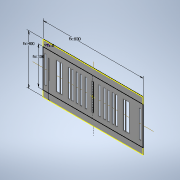
# Autodesk Inventor part: ferrite_layer_dex_1R1
Saved by Autodesk Inventor 2021 (Build 250183000, 183)
## iProperties
Created: 2021-01-27
Part Number: ferrite_layer_dex_1R1
Material: Generic
Document SubType Name: Modeling
Designer: pduy110
Density: 1 g/cm^3
Appearance: Smooth - Medium Gray
track_length: 800.000 mm
track_width: 300.000 mm
layer_width: 400.000 mm
ferrite_length: 218.000 mm
layer_length: 800.000 mm
real_sheet_width: 500.000 mm
ferrite_width: 15.000 mm
ferrite_height: 8.000 mm
number_of_ferrites: 7.000 ul
edge_gap_distance: 14.500 mm
parameter_2: 30.000 mm
parameter_5: 126.000 mm
parameter_6: 120.000 mm
bolt_diameter: 8.000 mm
number_of_bolts: 5.000 ul
x_offset_for_bolts: 75.000 mm
y_offset_for_bolts: 175.000 mm
wire_diameter: 4.500 mm
distance_between_wires: 18.600 mm
distance_between_wires_edge: 8.250 mm
bend_radius_inner: 15.000 mm
bend_radius_outer: 18.500 mm
wall_length: 800.000 mm
wall_width: 50.000 mm
wall_thickness: 25.000 mm
Author: pduy110
Autodesk Inventor part; units mm, degrees
ref_plane "YZ Plane" through (0, 0, 0) normal (1, 0, 0) x (0, 1, 0)
ref_plane "XZ Plane" through (0, 0, 0) normal (0, 1, 0) x (-1, 0, 0)
ref_plane "XY Plane" through (0, 0, 0) normal (0, 0, 1) x (1, 0, 0)
sketch "ferrite_layer_outline_sketch" plane through (0, 0, 0) normal (0, 0, 1) x (1, 0, 0)
  line L0 (-400, 200) -> (400, 200)
  line L1 (400, 200) -> (400, -200)
  line L2 (400, -200) -> (-400, -200)
  line L3 (-400, -200) -> (-400, 200)
  line L4 (0, 200) -> (0, -200) construction
  line L5 (0, 136.1953) -> (0, -273.5408) construction
  line L6 (0, 200) -> (0, -200)
  point P0 (0, 0)
  point P1 (0, 0)
  point P2 (0, 0)
  dimension "d85" = 800
  dimension "d86" = 400
  constraints: 14 end point, 4 midpoint, 2 parallel, 2 point on line, 1 coincident, 1 collinear, 1 horizontal, 1 perpendicular
  measures "d85" distance between parallel lines of L1 L3
  measures "d86" distance between parallel lines of L2 L0
extrude "Sheet Extrude" add sketch "ferrite_layer_outline_sketch" along normal blind 4
ref_plane "acrylic_sheet_plane" through (0, 0, 4) normal (0, 0, 1) x (1, 0, 0)
sketch "Sketch4" plane through (0, 0, 4) normal (0, 0, 1) x (1, 0, 0)
  line L0 (-385.5, 109) -> (-370.5, 109)
  line L1 (-370.5, 109) -> (-370.5, -109)
  line L2 (-370.5, -109) -> (-385.5, -109)
  line L3 (-385.5, -109) -> (-385.5, 109)
  line L4 (-12.6534, 0) -> (47.471, 0)
  line L5 (-400, 200) -> (-400, -200) projected
  line L6 (400, 200) -> (-400, 200) projected
  line L7 (-400, -200) -> (400, -200) projected
  point P0 (0, 0)
  point P1 (-385.5, 0)
  point P2 (-400, 0)
  dimension "d43" = 15
  dimension "d44" = 218
  dimension "d45" = 14.5
  constraints: 10 end point, 2 horizontal, 2 parallel, 2 point on line, 1 midpoint, 1 perpendicular, 2 other
  measures "d43" distance between parallel lines of L1 L3
  measures "d44" distance between parallel lines of L2 L0
extrude "Extrusion9" cut sketch "Sketch4" against normal through all
pattern_linear "Rectangular Pattern 7 fer" count 7 spacing 126 along (1, 0, 0) of "Extrusion9"
pattern_linear "Rectangular Pattern 8 fer" count 8 spacing 108 along (1, 0, 0) of "Extrusion9"
pattern_linear "pattern_test_#_of_ferrites 9 fer" count 9 spacing 94.5 along (1, 0, 0) of "Extrusion9"
pattern_linear "Rectangular Pattern 10 fer" [suppressed]
pattern_linear "Rectangular Pattern 13" [suppressed]
sketch "dimension_layout_sketch" plane through (0, 0, 4) normal (0, 0, 1) x (1, 0, 0)
  line L0 (-400, 200) -> (-400, -200) projected
  line L1 (400, -200) -> (400, 200) projected
  line L2 (400, 200) -> (-400, 200) projected
  line L3 (-400, -200) -> (400, -200) projected
  line L4 (-400, 150) -> (400, 150)
  line L5 (400, 150) -> (400, -150)
  line L6 (400, -150) -> (-400, -150)
  line L7 (-400, -150) -> (-400, 150)
  line L8 (0, 150) -> (0, -150) construction
  line L9 (-400, 200) -> (-400, -200) construction
  circle A0 centre (-359.2579, 182.7315) radius 4
  point P0 (0, 0)
  dimension "d87" = 300
  dimension "d88" = 8
  constraints: 10 end point, 3 midpoint, 2 parallel, 1 centre point, 1 collinear, 1 horizontal, 1 perpendicular, 1 other
  measures "d87" distance between parallel lines of L6 L4
  measures "d88" diameter of A0
sketch "wire_guide_layout_sketch" plane through (0, 0, 4) normal (0, 0, 1) x (1, 0, 0)
  line L0 (-400, -200) -> (400, -200) projected
  line L1 (-356.5, 92.3814) -> (-350, 92.3814)
  line L2 (-350, 92.3814) -> (-350, -200)
  line L3 (-350, -200) -> (-356.5, -200)
  line L4 (-356.5, -200) -> (-356.5, 92.3814)
  line L5 (-400, 200) -> (-400, -200) projected
  line L6 (-385.5, 109) -> (-370.5, 109) projected
  line L7 (-350, -60) -> (-345.5, -60)
  line L8 (-345.5, -60) -> (-345.5, -200)
  line L9 (-345.5, -200) -> (-350, -200)
  point P0 (0, 0)
  dimension "d89" = 43.5
  dimension "d90" = 6.5
  dimension "d91" = 140
  dimension "d92" = 4.5
  constraints: 14 end point, 3 point on line, 2 horizontal, 2 parallel, 2 perpendicular, 1 collinear
  measures "d89" distance between parallel lines of L5 L4
  measures "d90" distance between parallel lines of L4 L2
  measures "d91" distance between parallel lines of L0 L7
  measures "d92" distance between parallel lines of L2 L8
extrude "wire_guide Cut" cut sketch "wire_guide_layout_sketch" against normal through all
equation "\"d85\" = track_length"
equation "\"d86\" = layer_width"
equation "\"d43\" = ferrite_width"
equation "\"d44\" = ferrite_length"
equation "\"d45\" = edge_gap_distance"
equation "\"d50\" = parameter_5"
equation "\"d62\" = test_parameter_5"
equation "\"d87\" = track_width"
equation "\"d88\" = bolt_diameter"
equation "\"track_length\" = 800"
equation "\"track_width\" = 300"
equation "\"edge_gap_distance\" = 14.5"
equation "\"ferrite_length\" = 218"
equation "\"ferrite_width\" = 15"
equation "\"number_of_ferrites\" = 7"
equation "\"acrylic_sheet_8mm\" = 8"
equation "\"layer_width\" = 400"
equation "\"bolt_diameter\" = 8"
equation "\"layer_length\" = 800"
equation "\"real_sheet_width\" = 500"
equation "\"ferrite_height\" = 8"
equation "\"parameter_2\" = 30"
equation "\"parameter_6\" = 120"
equation "\"number_of_bolts\" = 5"
equation "\"x_offset_for_bolts\" = 75"
equation "\"y_offset_for_bolts\" = 175"
equation "\"wire_diameter\" = 4.5"
equation "\"distance_between_wires\" = -1.2 * wire_diameter + 0.2 * parameter_6"
equation "\"distance_between_wires_edge\" = -1.5 * wire_diameter + 0.5 * parameter_2"
equation "\"bend_radius_inner\" = 15"
equation "\"wall_length\" = track_length"
equation "\"wall_width\" = -0.5 * track_width + 0.5 * layer_width"
equation "\"wall_thickness\" = 25"
equation "\"parameter_5\" = 126"
equation "\"test_parameter_5\" = 94.5"
body "Solid8"
